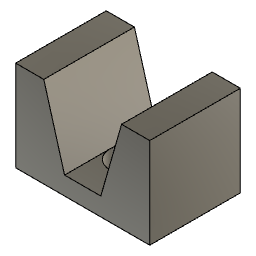
SensorShell (Autodesk Fusion 360 design; units mm, degrees)
Autodesk Fusion 360 part; units mm, degrees
note: some values were not read from the file. Chosen so that the rebuilt part matches the saved one: which face or edge a step refers to.
sketch "Sketch1" plane through (0, 0, 0) normal (0, 1, 0) x (1, 0, 0) in component "Sensor Shell"
  line L0 (0, 0) -> (0, -5)
  line L1 (0, -5) -> (-5, -5)
  line L2 (0, 0) -> (-16.5, 0)
  line L3 (-16.5, 0) -> (-16.5, -25)
  line L4 (-16.5, -25) -> (-10.73, -25)
  line L5 (-10.73, -25) -> (-5, -5)
  dimension "d12" = 5
  dimension "d13" = 5
  dimension "d14" = 16.5
  dimension "d15" = 25
  dimension "d17" = 5.77
  constraint coincident L0.start L2.start
  constraint vertical L0
  constraint perpendicular L0 L1
  constraint perpendicular L0 L2
  constraint perpendicular L2 L3
  constraint perpendicular L3 L4
  measures "d12" distance of L0.start L0.end
  measures "d13" distance of L0.end L1.end
  measures "d14" distance of L0.start L2.end
  measures "d15" distance of L2.end L3.end
  measures "d17" distance of L3.end L4.end
extrude "Extrude1" add sketch "Sketch1" along normal blind 25 makes body 1 in component "Sensor Shell"
mirror "MirrorComponent1" about plane through (0, 0, 0) normal (0, 0, 1) of bodies 1 makes body 2 in component "Sensor Shell(Mirror)"
combine "Combine1" operation add target body 1 tool bodies 2 body 2 seen with x (-1, 0, 0) y (0, 1, 0) z (0, 0, -1) at (0, 0, 0) in component "Sensor Shell"
hole "Hole1" at (0, 12.5, 5) direction (0, 0, -1) diameter 10 depth 9 tip angle 180 bodies 1 in component "Sensor Shell"
hole "Hole2" at (-13, 12.5, 0) direction (0, 0, 1) diameter 1.775 depth 3 tip angle 180 bodies 1 in component "Sensor Shell"
thread "Thread1" "ISO Metric profile 2.2 M2.2x0.45 6H" in component "Sensor Shell"
hole "Hole3" at (13, 12.5, 0) direction (0, 0, 1) diameter 1.775 depth 3 tip angle 180 bodies 1 in component "Sensor Shell"
thread "Thread2" "ISO Metric profile 2.2 M2.2x0.45 6H" in component "Sensor Shell"
move_face "OffsetFaces1" offset 2 1 faces at (16.5, 16.6667, 16.6667) on bodies 1 in component "Sensor Shell"
move_face "OffsetFaces2" offset 2 1 faces at (-16.5, 16.6667, 16.6667) on bodies 1 in component "Sensor Shell"
component "Sensor Shell" placed x (1, 0, 0) y (0, 1, 0) z (0, 0, 1) at (0, 0, 0)
component "Sensor Shell(Mirror)" placed x (-1, 0, 0) y (0, 1, 0) z (0, 0, -1) at (0, 0, 0)
